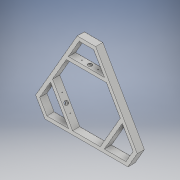
# Autodesk Inventor part: Frame
Saved by Autodesk Inventor 2018 (Build 220112000, 112)
## iProperties
Created: 2020-03-24
Part Number: Frame
Material: Generic
Document SubType Name: Modeling
Designer: maste
Density: 1 g/cm^3
Appearance: Default
Author: maste
Autodesk Inventor part; units mm, degrees
ref_plane "YZ Plane" through (0, 0, 0) normal (1, 0, 0) x (0, 1, 0)
ref_plane "XZ Plane" through (0, 0, 0) normal (0, 1, 0) x (-1, 0, 0)
ref_plane "XY Plane" through (0, 0, 0) normal (0, 0, 1) x (1, 0, 0)
sketch "Sketch1" plane through (0, 0, 0) normal (0, 0, 1) x (1, 0, 0)
  line L0 (0, 0) -> (254, 0)
  line L1 (254, 0) -> (177.8, 131.982272)
  line L2 (0, 0) -> (76.2, 131.982272)
  line L3 (0, 0) -> (152.4, 0) construction
  line L4 (76.2, 131.982272) -> (177.8, 131.982272)
  line L5 (0, 0) -> (254, 0) construction
  line L6 (127, 151.835687) -> (127, -477.263394) construction
  line L7 (61.535303, 157.382272) -> (-43.994091, -25.4)
  line L8 (-43.994091, -25.4) -> (297.994091, -25.4)
  line L9 (297.994091, -25.4) -> (192.464697, 157.382272)
  line L10 (192.464697, 157.382272) -> (61.535303, 157.382272)
  line L11 (453.797045, -408.646815) -> (-63.5, -109.985226) construction
  line L12 (-199.797045, -408.646815) -> (453.797045, -31.294091) construction
  line L13 (0, -439.940905) -> (-127, -219.970453)
  line L14 (0, -439.940905) -> (-127, -219.970453) construction
  line L15 (-127, -219.970453) -> (-203.2, -351.952724)
  line L16 (-127, -169.170453) -> (-232.529394, -351.952724)
  line L17 (43.994091, -465.340905) -> (-127, -169.170453)
  line L18 (-194.993562, -405.873522) -> (349.822223, -91.323982) construction
  line L19 (-152.4, -439.940905) -> (-203.2, -351.952724)
  line L20 (-232.529394, -351.952724) -> (-167.064697, -465.340905)
  line L21 (0, -439.940905) -> (-152.4, -439.940905)
  line L22 (-167.064697, -465.340905) -> (43.994091, -465.340905)
  line L23 (0, -439.940905) -> (-76.2, -307.958634) construction
  line L24 (381, -219.970453) -> (254, -439.940905)
  line L25 (381, -219.970453) -> (254, -439.940905) construction
  line L26 (254, -439.940905) -> (406.4, -439.940905)
  line L27 (210.005909, -465.340905) -> (421.064697, -465.340905)
  line L28 (381, -169.170453) -> (210.005909, -465.340905)
  line L29 (448.993562, -405.873522) -> (-95.822223, -91.323982) construction
  line L30 (457.2, -351.952724) -> (406.4, -439.940905)
  line L31 (421.064697, -465.340905) -> (486.529394, -351.952724)
  line L32 (381, -219.970453) -> (457.2, -351.952724)
  line L33 (486.529394, -351.952724) -> (381, -169.170453)
  line L34 (381, -219.970453) -> (304.8, -351.952724) construction
  point P0 (127, -219.970453)
  dimension "d0" = 254
  dimension "d1" = 152.4
  dimension "d2" = 60
  dimension "d3" = 152.4
  dimension "d4" = 60
  dimension "d11" = 25.4
  dimension "d22" = 360
  constraints: 70 end point, 3 horizontal, 1 equal length, 1 midpoint, 1 point on line, 1 vertical, 73 other
  measures "d0" distance of L0.start L0.end
  measures "d1" distance of L0.end L1.end
  measures "d2" angle of L1 L0
  measures "d3" distance of L0.start L2.end
  measures "d4" angle of L3 L2
  measures "d11" distance between parallel lines of L2 L7
extrude "Extrusion1" add sketch "Sketch1" along normal blind 50.8
sketch "Sketch2" plane through (0, 0, 50.8) normal (0, 0, 1) x (1, 0, 0)
  line L0 (61.535303, 157.382272) -> (-43.994091, -25.4)
  line L1 (-43.994091, -25.4) -> (-127.322087, -169.728323)
  line L2 (-127, -219.970453) -> (0, -439.940905)
  line L3 (0, 0) -> (-127, -219.970453)
  line L4 (-127, -169.170453) -> (43.994091, -465.340905)
  line L5 (-127, -219.970453) -> (-127, -169.170453)
  line L6 (0, 0) -> (76.2, 131.982272)
  line L7 (0, 0) -> (-43.994091, -25.4)
  line L8 (254, 0) -> (0, 0)
  line L9 (-43.994091, -25.4) -> (297.994091, -25.4)
  line L10 (254, 0) -> (297.994091, -25.4)
  line L11 (381, -169.170453) -> (210.005909, -465.340905)
  line L12 (297.994091, -25.4) -> (381, -169.170453)
  line L13 (254, -439.940905) -> (381, -219.970453)
  line L14 (381, -169.170453) -> (381, -219.970453)
  line L15 (381, -219.970453) -> (254, 0)
  line L16 (254, -439.940905) -> (210.005909, -465.340905)
  line L17 (210.005909, -465.340905) -> (43.994091, -465.340905)
  line L18 (43.994091, -465.340905) -> (0, -439.940905)
  line L19 (0, -439.940905) -> (254, -439.940905)
  constraints: 24 end point, 3 perpendicular, 2 parallel, 2 vertical, 1 collinear
extrude "Extrusion2" add sketch "Sketch2" against normal blind 50.8 contours L9 L3 L4 L1 | L7 L3 L9 | L4 L3 L5 | L10 L9 L15 | L9 L12 L11 L15 | L11 L14 L15
sketch "Sketch3" plane through (0, 0, 50.8) normal (0, 0, 1) x (1, 0, 0)
  line L0 (43.994091, -465.340905) -> (-167.064697, -465.340905)
  line L1 (421.064697, -465.340905) -> (210.005909, -465.340905)
  line L2 (43.994091, -465.340905) -> (210.005909, -465.340905)
  line L3 (381, -219.970453) -> (254, -439.940905)
  line L4 (210.005909, -465.340905) -> (254, -439.940905)
  line L5 (-152.4, -439.940905) -> (0, -439.940905)
  line L6 (254, -439.940905) -> (0, -439.940905)
  line L7 (0, -439.940905) -> (43.994091, -465.340905)
  point P0 (0, 0)
  constraints: 8 end point, 1 collinear, 1 horizontal
extrude "Extrusion3" add sketch "Sketch3" against normal blind 50.8
sketch "Sketch4" plane through (-14.664697, -25.4, 0) normal (0, -1, 0) x (1, 0, 0)
  line L0 (0, 0) -> (283.329394, 0) construction
  line L1 (141.664697, 0) -> (141.664697, 25.4) construction
  line L2 (141.664697, 0) -> (167.064697, 0) construction
  circle A0 centre (141.664697, 25.4) radius 14.2875
  line L3 (141.664697, 25.4) -> (198.814697, 25.4) construction
  line L4 (141.664697, 25.4) -> (84.514697, 25.4) construction
  circle A1 centre (198.814697, 25.4) radius 2.4892
  circle A2 centre (84.514697, 25.4) radius 2.4892
  point P0 (14.664697, 0)
  dimension "d30" = 25.4
  dimension "d31" = 90
  dimension "d32" = 28.575
  dimension "d34" = 57.15
  dimension "d35" = 57.15
  dimension "d36" = 4.9784
  dimension "d37" = 4.9784
  constraints: 8 end point, 3 centre point, 3 coincident, 3 horizontal, 1 midpoint, 1 perpendicular, 1 vertical
  measures "d30" distance of L1.start L1.end
  measures "d31" angle of L2 L1
  measures "d32" diameter of A0
  measures "d34" distance of L3.start L3.end
  measures "d35" distance of L3.start L4.end
  measures "d36" diameter of A1
  measures "d37" diameter of A2
shell "Shell1" thickness 1.5875 removed faces 0
extrude "Extrusion4" cut sketch "Sketch4" against normal blind 25.4
sketch "Sketch5" plane through (-112.335303, -194.570453, 50.8) normal (0.8660254, 0.5, 0) x (0, 0, -1)
  line L0 (50.8, 0) -> (50.8, -283.329394) construction
  line L1 (50.8, -141.664697) -> (25.4, -141.664697) construction
  line L2 (50.8, -141.664697) -> (76.2, -141.664697) construction
  line L3 (25.4, -141.664697) -> (25.4, -84.514697) construction
  line L4 (25.4, -141.664697) -> (25.4, -198.814697) construction
  circle A0 centre (25.4, -198.814697) radius 2.4892
  circle A1 centre (25.4, -84.514697) radius 2.4892
  circle A2 centre (25.4, -141.664697) radius 14.2875
  point P0 (50.8, 112.335303)
  dimension "d40" = 25.4
  dimension "d41" = 180
  dimension "d42" = 57.15
  dimension "d43" = 57.15
  dimension "d44" = 4.9784
  dimension "d45" = 4.9784
  dimension "d46" = 28.575
  constraints: 8 end point, 3 centre point, 3 coincident, 2 perpendicular, 1 collinear, 1 horizontal, 1 midpoint, 1 vertical
  measures "d40" distance of L1.start L1.end
  measures "d41" angle of L1 L2
  measures "d42" distance of L1.end L3.end
  measures "d43" distance of L1.end L4.end
  measures "d44" diameter of A0
  measures "d45" diameter of A1
  measures "d46" diameter of A2
extrude "Extrusion5" cut sketch "Sketch5" against normal blind 25.4
body "Solid1"
